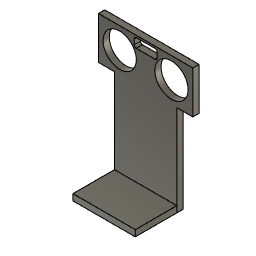
US_sensor_mount v1 (Autodesk Fusion 360 design; units mm, degrees)
Autodesk Fusion 360 part; units mm, degrees
sketch "Sketch3" plane through (0, 0, 0) normal (0, 1, 0) x (1, 0, 0)
  circle A0 centre (12.4, 0) radius 8
  line L0 (-22.7, 10.2) -> (-22.7, -10.2)
  line L1 (-22.7, -10.2) -> (22.7, -10.2)
  line L2 (22.7, -10.2) -> (22.7, 10.2)
  line L3 (22.7, 10.2) -> (-22.7, -10.2) construction
  line L4 (-22.7, 10.2) -> (22.7, -10.2) construction
  circle A1 centre (-12.5, 0) radius 8
  line L5 (4.5, -4.75) -> (-4.5, -4.75)
  line L6 (-5.5, -5.75) -> (-5.5, -8.25)
  line L7 (-4.5, -9.25) -> (4.5, -9.25)
  line L8 (5.5, -8.25) -> (5.5, -5.75)
  line L9 (5.5, -4.75) -> (-5.5, -9.25) construction
  line L10 (-5.5, -4.75) -> (5.5, -9.25) construction
  arc A2 (-5.5, -8.25) -> (-4.5, -9.25) centre (-4.5, -8.25) ccw
  arc A3 (4.5, -9.25) -> (5.5, -8.25) centre (4.5, -8.25) ccw
  arc A4 (5.5, -5.75) -> (4.5, -4.75) centre (4.5, -5.75) ccw
  arc A5 (-4.5, -4.75) -> (-5.5, -5.75) centre (-4.5, -5.75) ccw
  line L11 (15.0179, 10.2) -> (15.0179, 54)
  line L12 (15.0179, 54) -> (-14.9821, 54)
  line L13 (-14.9821, 54) -> (-14.9821, 10.2)
  line L14 (22.7, 10.2) -> (15.0179, 10.2)
  line L15 (-14.9821, 10.2) -> (-22.7, 10.2)
  point P0 (0, -7)
  dimension "d8" = 16
  dimension "d10" = 45.4
  dimension "d11" = 20.4
  dimension "d12" = 16
  dimension "d13" = 11
  dimension "d14" = 4.5
  dimension "d15" = 1
  dimension "d16" = 1
  dimension "d17" = 30
  dimension "d18" = 43.8
  constraint perpendicular L0 L14
  constraint parallel L1 L14
  constraint parallel L0 L2
  constraint horizontal L14
  constraint coincident L3 origin
  constraint coincident L4 origin
  constraint perpendicular L5 L6
  constraint parallel L5 L7
  constraint parallel L6 L8
  constraint horizontal L5
  constraint coincident L9 P0
  constraint coincident L10 P0
  constraint coincident L9.end L7
  constraint coincident L9.end L6
  constraint tangent L7 A2
  constraint tangent L6 A2
  constraint coincident L10.end L7
  constraint coincident L10.end L8
  constraint tangent L7 A3
  constraint tangent L8 A3
  constraint equal A2 A3
  constraint coincident L9.start L5
  constraint coincident L9.start L8
  constraint tangent L5 A4
  constraint tangent L8 A4
  constraint equal A2 A4
  constraint coincident L10.start L6
  constraint coincident L10.start L5
  constraint tangent L6 A5
  constraint tangent L5 A5
  constraint vertical L11
  constraint horizontal L12
  constraint vertical L13
  constraint coincident L13.end L14
  measures "d8" diameter of A0
  measures "d10" distance of L0.end L1.end
  measures "d11" distance of L0.start L0.end
  measures "d12" diameter of A1
  measures "d13" distance of L9.end L10.end
  measures "d14" distance of L10.start L9.end
  measures "d15" radius of A2
  measures "d16" radius of A5
  measures "d17" distance of L13.end L11.start
  measures "d18" distance of L13.end L12.end
sketch "Sketch4" plane through (0, 0, 0) normal (0, 1, 0) x (1, 0, 0)
  line L0 (-15, 54) -> (15, 54)
  line L1 (15, 54) -> (15, 51)
  line L2 (15, 51) -> (-15, 51)
  line L3 (-15, 51) -> (-15, 54)
  constraint horizontal L0
  constraint vertical L1
  constraint horizontal L2
  constraint vertical L3
extrude "Extrude1" add sketch "Sketch3" along normal blind 3
extrude "Extrude2" add sketch "Sketch4" against normal blind 20
sketch "Sketch1" plane through (0, 0, 0) normal (0, 1, 0) x (1, 0, 0)
sketch "Sketch2" plane through (0, 0, 0) normal (0, 1, 0) x (1, 0, 0)
